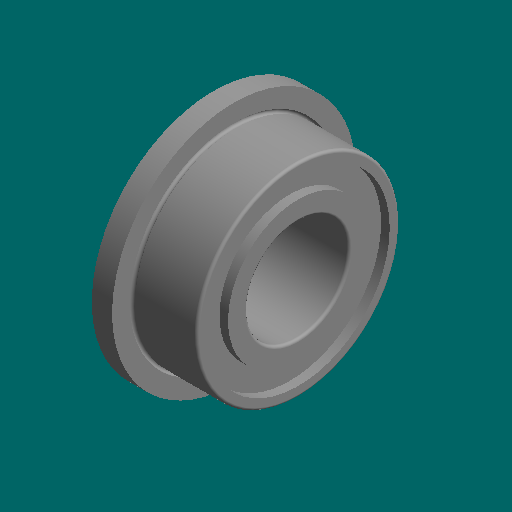
# Autodesk Inventor part: FL673ZZ
Saved by Autodesk Inventor 2023 (Build 270158000, 158)
## iProperties
Category: PARTsolutions
Company: MISUMI
Part Number: FL673ZZ
Material: 一般
Catalog Web Link: www.cadenas.de
Description: FL6 _ _ ZZ, FL6 _ _ AZZ, SFL6 _ _ ZZ, SFL6 _ _ AZZ, MFL1 _ _ ZZ, SMFL1 _ _ ZZ-Flanged Ball Bearings (Small Diameter, Deep Groove) - Double Shield Type
Vendor: MISUMI
Document SubType Name: Modeling
Designer: partserver
Manufacturer: MISUMI
Mass: 0.0553621 g
Surface Area: 1.5828 cm^2
Volume: 0.0553621 cm^3
Density: 1 g/cm^3
Appearance: PSOLRGB-175-175-175
PSOL_IDENT_0: {$CADENAS_DATA\23d-libs\misumi\metric\12_bearing_holders\sfl608zz.prj},228 {VTYP=3D},{NB=FL673ZZ},{L
PSOL_IDENT_1: INA=FL673ZZ},{NN=FL6 _ _ ZZ, FL6 _ _ AZZ, SFL6 _ _ ZZ, SFL6 _ _ AZZ, MFL1 _ _ ZZ, SMFL1 _ _ ZZ},{DAT
PSOL_IDENT_2: E=09.09.2019 15:26:56},{GEOMDATE=16.08.2017 04:27:24},{VERSION=},{LINEID=10},{WBVAR=MAT},{WBNUMERIC=
PSOL_IDENT_3: }  {NB=FL673ZZ},{LINA=FL673ZZ},{KT=DUMMY},{PN=FL673ZZ},{MAT=},{MAT1= '', '52100 Bearing Steel', 'S',
PSOL_IDENT_4: '440C Stainless Steel'},{BN=673ZZ},{DD=3.0},{AA=1.9900},{BB=0.3000},{C1=0.5750},{D=6},{B=2.5},{D1=7
PSOL_IDENT_5: .2},{C=0.6},{RR=0.08},{CR=242},{COR=94},{CRS=242},{CRSS=178},{CORS=94},{CORSS=59},{DS=3.60},{R=0.08}
PSOL_IDENT_6: ,{MASS=0.26},{MAT11=1},{MMMM=}
NB: FL673ZZ
NN: FL6 _ _ ZZ, FL6 _ _ AZZ, SFL6 _ _ ZZ, SFL6 _ _ AZZ, MFL1 _ _ ZZ, SMFL1 _ _ ZZ
NT: Flanged Ball Bearings (Small Diameter, Deep Groove) - Double Shield Type
NBSYN: $PN.
LINA: FL673ZZ
CATALOG: Misumi
PN: FL673ZZ
MAT: 52100 Bearing Steel
BN: 673ZZ
DD: 3
D: 6
B: 2.5
D1: 0
C: 0.6
RR: 0.08
CR: 242
COR: 94
DS: 3.6
R: 0.08
MASS: 0.26
SUPPLIER: MISUMI
ARTICLENO: FL673ZZ
BOMINFO: FL673ZZ
CREATOR: CADENAS GmbH
Title: FL673ZZ
Author: Cadenas PARTsolutions
Comments: Flanged Ball Bearings (Small Diameter, Deep Groove) - Double Shield Type
Autodesk Inventor part; units mm, degrees
ref_plane "YZ Plane" through (0, 0, 0) normal (1, 0, 0) x (0, 1, 0)
ref_plane "XZ Plane" through (0, 0, 0) normal (0, 1, 0) x (-1, 0, 0)
ref_plane "XY Plane" through (0, 0, 0) normal (0, 0, 1) x (1, 0, 0)
sketch "Sketch_1" plane through (0, 0, 0) normal (0, 0, 1) x (1, 0, 0)
  line L0 (6, 0) -> (-6, 0)
  arc A0 (0, 1.58) -> (0.08, 1.5) centre (0.08, 1.58) ccw
  line L1 (0.08, 1.5) -> (2.42, 1.5)
  arc A1 (2.42, 1.5) -> (2.5, 1.58) centre (2.42, 1.58) ccw
  line L2 (2.5, 1.58) -> (2.5, 2.075)
  line L3 (2.5, 2.075) -> (2.245, 2.075)
  line L4 (2.245, 2.075) -> (2.245, 2.7)
  line L5 (2.245, 2.7) -> (2.5, 2.7)
  line L6 (2.5, 2.7) -> (2.5, 3.6)
  line L7 (2.5, 3.6) -> (1.9, 3.6)
  line L8 (1.9, 3.6) -> (1.9, 3.08)
  arc A2 (1.82, 3) -> (1.9, 3.08) centre (1.9, 3) ccw
  line L9 (1.82, 3) -> (0.08, 3)
  arc A3 (0.08, 3) -> (0, 2.92) centre (0.08, 2.92) ccw
  line L10 (0, 2.92) -> (0, 2.7)
  line L11 (0, 2.7) -> (0.255, 2.7)
  line L12 (0.255, 2.7) -> (0.255, 2.075)
  line L13 (0.255, 2.075) -> (0, 2.075)
  line L14 (0, 2.075) -> (0, 1.58)
  constraints: 30 end point, 8 point on circle, 4 centre point
revolve "Revolution1" add sketch "Sketch_1" angle 360 about axis through (6, 0, 0) along (1, 0, 0)
ref_plane "to_housing_XY" through (0, 0, 0) normal (1, 0, 0) x (0, 0, -1)
ref_plane "to_housing_YZ" through (0, 0, 0) normal (0, 0, -1) x (0, 1, 0)
ref_plane "to_housing_ZX" through (0, 0, 0) normal (0, 1, 0) x (1, 0, 0)
body "Solid1"
